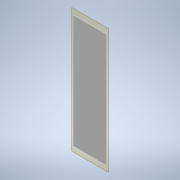
# Autodesk Inventor part: placa superior
Saved by Autodesk Inventor 2021 (Build 250183000, 183)
## iProperties
Created: 2021-03-18
Part Number: placa superior
Material: Stainless Steel
Document SubType Name: Modeling
Designer: andre
Density: 8 g/cm^3
Appearance: Semi-Polished
Author: andre
Autodesk Inventor part; units mm, degrees
ref_plane "YZ Plane" through (0, 0, 0) normal (1, 0, 0) x (0, 1, 0)
ref_plane "XZ Plane" through (0, 0, 0) normal (0, 1, 0) x (-1, 0, 0)
ref_plane "XY Plane" through (0, 0, 0) normal (0, 0, 1) x (1, 0, 0)
ref_plane "Work Plane1" through (0, 0, 0) normal (0, 0, 1) x (1, 0, 0)
sketch "Sketch1" plane through (0, 0, 0) normal (0, 0, 1) x (1, 0, 0)
  line L0 (-450, 1150) -> (-450, -1150) projected
  line L1 (-450, -1150) -> (450, -1150) projected
  line L2 (450, -1150) -> (450, 1150) projected
  line L3 (450, 1150) -> (-450, 1150) projected
  line L4 (-225, 600) -> (-225, 1050) projected
  line L5 (-225, 600) -> (-225, 500) projected
  line L6 (-225, 500) -> (-225, 50) projected
  line L7 (-225, 50) -> (-225, -50) projected
  line L8 (-225, -500) -> (-225, -50) projected
  line L9 (-225, -600) -> (-225, -500) projected
  line L10 (-225, 1150) -> (-225, 1050) projected
  line L11 (-225, -1050) -> (-225, -600) projected
  line L12 (-225, -1150) -> (-225, -1050) projected
  point P0 (0, 0)
extrude "Extrusion1" add sketch "Sketch1" along normal blind 6.35 contours L3 L2 L1 L12 L11 L9 L8 L7 L6 L5 L4 L10
body "Solid1"
